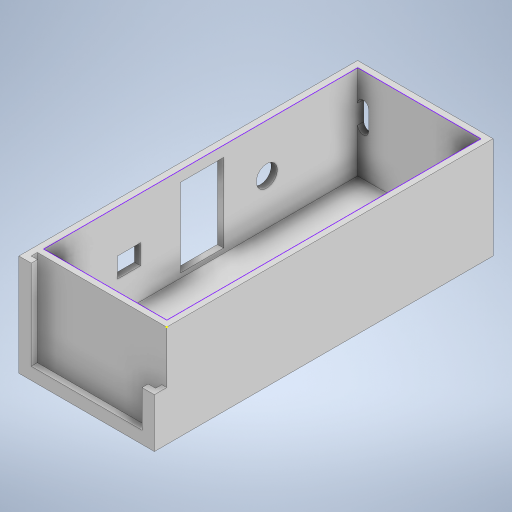
# Autodesk Inventor part: roller_box_new03_10_2025
Saved by Autodesk Inventor 2024.2 (Build 282272000, 272)
## iProperties
Created: 2025-08-30
Part Number: roller_box_new03_10_2025
Material: Типовые
Document SubType Name: Modeling
Designer: winds
Density: 1 g/cm^3
Appearance: По умолчанию
Author: winds
Autodesk Inventor part; units mm, degrees
ref_plane "YZ Plane" through (0, 0, 0) normal (1, 0, 0) x (0, 1, 0)
ref_plane "XZ Plane" through (0, 0, 0) normal (0, 1, 0) x (-1, 0, 0)
ref_plane "XY Plane" through (0, 0, 0) normal (0, 0, 1) x (1, 0, 0)
sketch "внешние размеры" plane through (0, 0, 0) normal (0, 1, 0) x (-1, 0, 0)
  line L0 (0, 0) -> (44, 0)
  line L1 (44, 0) -> (44, -106)
  line L2 (44, -106) -> (0, -106)
  line L3 (0, -106) -> (0, 0)
  dimension "d0" = 44
  dimension "d1" = 106
  constraints: 8 end point, 2 parallel, 1 horizontal, 1 perpendicular
  measures "d0" distance of L0.start L0.end
  measures "d1" distance between parallel lines of L0 L2
extrude "Выдавливание1" add sketch "внешние размеры" along normal blind 33
sketch "внутренние размеры" plane through (0, 33, 0) normal (0, 1, 0) x (1, 0, 0)
  line L0 (-42, 2) -> (-2, 2)
  line L1 (-2, 2) -> (-2, 104)
  line L2 (-2, 104) -> (-42, 104)
  line L3 (-42, 104) -> (-42, 2)
  point P0 (0, 0)
  constraints: 8 end point, 2 parallel, 1 horizontal, 1 perpendicular
extrude "Выдавливание2" cut sketch "внутренние размеры" against normal blind 30.5
sketch "перегородка" plane through (0, 2.5, 0) normal (0, 1, 0) x (1, 0, 0)
  line L0 (-42, 104) -> (-2, 104) projected
  line L1 (-20.5, 104) -> (-21.5, 104)
  line L2 (-21.5, 104) -> (-21.5, 54)
  line L3 (-21.5, 54) -> (-20.5, 54)
  line L4 (-20.5, 54) -> (-20.5, 104)
  line L5 (-2, 104) -> (-2, 2) projected
  line L6 (-42, 104) -> (-2, 104) projected
  point P0 (0, 0)
  point P1 (-22, 104)
  point P2 (-21, 54)
  dimension "d6" = 18.5
  dimension "d7" = 1
  dimension "d8" = 50
  constraints: 8 end point, 2 midpoint, 2 parallel, 1 horizontal, 1 perpendicular, 1 point on line
  measures "d6" distance between parallel lines of L4 L5
  measures "d7" distance between parallel lines of L4 L2
  measures "d8" vertical distance of point (-22, 104) point (-21, 54)
extrude "Выдавливание3" add sketch "перегородка" along normal blind 10
sketch "дисплей" plane through (-44, 0, -106) normal (-1, 0, 0) x (0, 0, 1)
  line L0 (45.5, 4) -> (59.5, 4)
  line L1 (59.5, 4) -> (59.5, 29.5)
  line L2 (59.5, 29.5) -> (45.5, 29.5)
  line L3 (45.5, 29.5) -> (45.5, 4)
  line L4 (0, 0) -> (0, 33) projected
  line L5 (0, 0) -> (106, 0) projected
  line L6 (0, 33) -> (106, 33) projected
  point P0 (0, 16.5)
  point P1 (59.5, 16.75)
  dimension "d21" = 25.5
  dimension "d22" = 14
  dimension "d23" = 45.5
  dimension "d24" = 4
  dimension "d25" = 3.5
  dimension "d125" = 59.5
  constraints: 8 end point, 2 midpoint, 2 parallel, 1 horizontal, 1 perpendicular
  measures "d21" distance of L2.end L0.start
  measures "d22" distance of L1.end L2.end
  measures "d23" distance between parallel lines of L4 L3
  measures "d24" distance between parallel lines of L5 L0
  measures "d25" distance between parallel lines of L6 L2
  measures "d125" horizontal distance of point (0, 16.5) point (59.5, 16.75)
extrude "Выдавливание4" cut sketch "дисплей" against normal blind 2.5
sketch "уф" plane through (-44, 0, -106) normal (-1, 0, 0) x (0, 0, 1)
  line L0 (80, 12.5) -> (72.5, 12.5)
  line L1 (72.5, 12.5) -> (72.5, 19)
  line L2 (72.5, 19) -> (80, 19)
  line L3 (80, 19) -> (80, 12.5)
  line L4 (106, 0) -> (106, 33) projected
  line L5 (0, 0) -> (106, 0) projected
  line L6 (0, 33) -> (106, 33) projected
  line L7 (0, 0) -> (0, 33) projected
  point P0 (80, 15.75)
  point P1 (72.5, 15.75)
  point P2 (0, 16.5)
  dimension "d28" = 7.5
  dimension "d29" = 6.5
  dimension "d30" = 26
  dimension "d31" = 12.5
  dimension "d32" = 14
  dimension "d126" = 72.5
  constraints: 8 end point, 3 midpoint, 2 parallel, 1 horizontal, 1 perpendicular
  measures "d28" distance of point (80, 15.75) point (72.5, 15.75)
  measures "d29" distance between parallel lines of L2 L0
  measures "d30" distance between parallel lines of L4 L3
  measures "d31" distance between parallel lines of L5 L0
  measures "d32" distance between parallel lines of L6 L2
  measures "d126" horizontal distance of point (0, 16.5) L1.end
extrude "Выдавливание5" cut sketch "уф" against normal blind 2.5 contours L0 L1 L2 L3
sketch "usb-c" plane through (0, 0, -106) normal (0, 0, -1) x (-1, 0, 0)
  line L0 (40.2, 24.8) -> (40.2, 15) construction
  line L1 (42, 4) -> (42, 29.5) projected
  line L2 (42, 23) -> (42, 16.8)
  line L3 (38.4, 16.8) -> (38.4, 23)
  arc A0 (42, 23) -> (38.4, 23) centre (40.2, 23) ccw
  arc A1 (38.4, 16.8) -> (42, 16.8) centre (40.2, 16.8) ccw
  line L4 (44, 0) -> (44, 33) projected
  line L5 (0, 0) -> (44, 0) projected
  point P0 (40.2, 19.9)
  point P1 (42, 19.9)
  point P2 (38.4, 19.9)
  point P3 (42, 16.8)
  point P4 (42, 23)
  dimension "d35" = 2
  dimension "d36" = 15
  dimension "d37" = 9.8
  dimension "d38" = 3.6
  constraints: 8 end point, 8 point on circle, 4 tangent, 3 midpoint, 2 centre point, 2 parallel, 2 point on line
  measures "d35" distance from line of L4 point (42, 19.9)
  measures "d36" distance from line of L5 point (40.2, 15)
  measures "d37" distance of point (40.2, 24.8) L0.end
  measures "d38" distance of point (38.4, 19.9) point (42, 19.9)
extrude "Выдавливание6" cut sketch "usb-c" against normal blind 2.5
sketch "stepper уши" plane through (0, 2.5, 0) normal (0, 1, 0) x (1, 0, 0)
  line L0 (-42, 2) -> (-42, 104) projected
  line L1 (-2, 2) -> (-42, 2) projected
  point P0 (0, 0)
  point P1 (-38.5, 5.5)
  point P2 (-15.5, 32)
  point P3 (-33, 24)
  point P4 (-33, 24)
  dimension "d41" = 3.5
  dimension "d42" = 3.5
  dimension "d43" = 26.5
  dimension "d44" = 30
  dimension "d45" = 35.0892
  dimension "d46" = 22
  dimension "d47" = 9
  dimension "d48" = 19.2419
  dimension "d49" = 19.3003
  constraints: 1 coincident
  measures "d41" distance from line of L0 point (-38.5, 5.5)
  measures "d42" distance from line of L1 point (-38.5, 5.5)
  measures "d43" distance from line of L0 point (-15.5, 32)
  measures "d44" distance from line of L1 point (-15.5, 32)
  measures "d45" distance of point (-15.5, 32) point (-38.5, 5.5)
  measures "d46" distance from line of L1 point (-33, 24)
  measures "d47" distance from line of L0 point (-33, 24)
  measures "d48" distance of point (-15.5, 32) point (-33, 24)
  measures "d49" distance of point (-33, 24) point (-38.5, 5.5)
hole "Отверстие2" at (-33, 2.5, -24) at (-15.5, 2.5, -32) at (-38.5, 2.5, -5.5) at (-33, 2.5, -24) direction (0, -1, 0) diameter 2.5 depth 2.5 tip angle 118
sketch "stepper ось" plane through (0, 2.5, 0) normal (0, 1, 0) x (1, 0, 0)
  circle A0 centre (-33, 24) radius 1.25 projected
  line L0 (-44, 0) -> (0, 0) projected
  line L1 (0, 0) -> (0, 106) projected
  dimension "d127" = 24
  dimension "d128" = 33
  constraints: 1 coincident
  measures "d127" distance from line of L0 point (-33, 24)
  measures "d128" distance from line of L1 point (-33, 24)
hole "Отверстие3" at (-33, 2.5, -24) direction (0, -1, 0) diameter 10 depth 2.5 tip angle 118
sketch "solar" plane through (0, 2.5, 0) normal (0, 1, 0) x (1, 0, 0)
  line L0 (-2, 104) -> (-2, 2) projected
  line L1 (-2, 2) -> (-8, 2)
  line L2 (-8, 2) -> (-8, 9.5)
  line L3 (-8, 9.5) -> (-2, 9.5)
  line L4 (-2, 9.5) -> (-2, 2)
  point P0 (0, 0)
  point P1 (-5, 2)
  point P2 (-5, 9.5)
  point P3 (-2, 9.5)
  dimension "d64" = 6
  dimension "d65" = 7.5
  constraints: 8 end point, 2 midpoint, 2 parallel, 1 horizontal, 1 perpendicular
  measures "d64" distance between parallel lines of L0 L2
  measures "d65" distance of point (-5, 2) point (-5, 9.5)
extrude "Выдавливание7" cut sketch "solar" against normal blind 2.5
sketch "кнопка" plane through (-44, 0, -106) normal (-1, 0, 0) x (0, 0, 1)
  line L0 (0, 0) -> (106, 0) projected
  line L1 (0, 0) -> (0, 33) projected
  point P0 (31.5, 17.3)
  dimension "d116" = 17.3
  dimension "d117" = 31.5
  measures "d116" distance from line of L0 point (31.5, 17.3)
  measures "d117" distance from line of L1 point (31.5, 17.3)
hole "Отверстие7" at (-44, 17.3, -74.5) direction (1, 0, 0) diameter 6.9 depth 2.5 tip angle 118
sketch "Эскиз25" plane through (-44, 0, -106) normal (-1, 0, 0) x (0, 0, 1)
  line L0 (106, 0) -> (106, 33) projected
  line L1 (106, 33) -> (110, 33)
  line L2 (110, 33) -> (110, 0)
  line L3 (110, 0) -> (106, 0)
  line L4 (106, 0) -> (106, 33)
  constraints: 8 end point, 2 parallel, 1 horizontal, 1 perpendicular
extrude "Выдавливание12" add sketch "Эскиз25" against normal blind 44
sketch "паз" plane through (-44, 0, -106) normal (-1, 0, 0) x (0, 0, 1)
  line L0 (106, 33) -> (108, 33)
  line L1 (108, 33) -> (108, 2)
  line L2 (108, 2) -> (106, 2)
  line L3 (106, 2) -> (106, 33)
  line L4 (110, 33) -> (110, 0) projected
  line L5 (108, 33) -> (110, 33)
  line L6 (110, 33) -> (110, 4)
  line L7 (110, 4) -> (108, 4)
  line L8 (108, 4) -> (108, 33)
  point P0 (106, 0)
  point P1 (107, 2)
  point P2 (107, 33)
  point P3 (109, 4)
  point P4 (109, 33)
  dimension "d133" = 31
  dimension "d134" = 29
  dimension "d135" = 2
  constraints: 16 end point, 4 midpoint, 4 parallel, 2 horizontal, 2 perpendicular, 2 point on line
  measures "d133" distance of point (107, 2) point (107, 33)
  measures "d134" distance of point (109, 4) point (109, 33)
  measures "d135" distance between parallel lines of L1 L3
extrude "Выдавливание13" cut sketch "паз" against normal blind 44
sketch "Эскиз27" plane through (0, 2.5, 0) normal (0, 1, 0) x (1, 0, 0)
  line L0 (-42, 104) -> (-2, 104) projected
  line L1 (-18, 60) -> (-17, 60)
  line L2 (-17, 60) -> (-17, 104)
  line L3 (-17, 104) -> (-18, 104)
  line L4 (-18, 104) -> (-18, 60)
  point P0 (0, 0)
  constraints: 8 end point, 2 parallel, 1 horizontal, 1 perpendicular, 1 point on line
extrude "Выдавливание14" add sketch "Эскиз27" along normal blind 3 draft -10
sketch "Эскиз28" plane through (0, 2.5, 0) normal (0, 1, 0) x (1, 0, 0)
  line L0 (-2, 104) -> (-2, 2) projected
  line L1 (-2, 18) -> (-10, 18)
  line L2 (-10, 18) -> (-10, 19)
  line L3 (-10, 19) -> (-2, 19)
  line L4 (-2, 19) -> (-2, 18)
  line L5 (-2, 104) -> (-2, 9.5) projected
  line L6 (-2, 27) -> (-10, 27)
  line L7 (-10, 27) -> (-10, 28)
  line L8 (-10, 28) -> (-2, 28)
  line L9 (-2, 28) -> (-2, 27)
  line L10 (-10, 28) -> (-11, 28)
  line L11 (-11, 28) -> (-11, 18)
  line L12 (-11, 18) -> (-10, 18)
  line L13 (-10, 18) -> (-10, 28)
  point P0 (0, 0)
  point P1 (-2, 19)
  constraints: 24 end point, 6 parallel, 3 horizontal, 3 perpendicular, 3 point on line
extrude "Выдавливание15" add sketch "Эскиз28" along normal blind 13.5 contours L0 L6 L7 L8 | L7 L13 L2 L12 L11 L10 | L0 L1 L2 L3
sketch "кнопка2" plane through (0, 2.5, 0) normal (0, 1, 0) x (1, 0, 0)
  circle A0 centre (-6, 23) radius 3.6
  line L0 (0, -4) -> (0, 106) projected
  line L1 (-2, 19) -> (-10, 19) projected
  point P0 (0, 0)
  dimension "d147" = 7.2
  dimension "d172" = 6
  dimension "d173" = 4
  constraints: 1 centre point
  measures "d147" diameter of A0
  measures "d172" distance from line of L0 A0.centre
  measures "d173" distance from line of A0.centre L1
hole "Отверстие9" at (-6, 2.5, -23) direction (0, -1, 0) diameter 7.2 depth 2.5 tip angle 118
sketch "Эскиз31" plane through (0, 2.5, 0) normal (0, 1, 0) x (1, 0, 0)
  line L0 (-2, 104) -> (-2, 2) projected
  line L1 (-2, 2) -> (-42, 2) projected
  line L2 (-2, 10) -> (-3, 10)
  line L3 (-3, 10) -> (-3, 2)
  line L4 (-3, 2) -> (-2, 2)
  line L5 (-2, 2) -> (-2, 10)
  point P0 (0, 0)
  constraints: 8 end point, 2 parallel, 2 point on line, 1 horizontal, 1 perpendicular
extrude "Выдавливание16" add sketch "Эскиз31" along normal blind 2
sketch "Эскиз32" plane through (-44, 4, 4) normal (0, 1, 0) x (1, 0, 0)
  line L0 (0, 0) -> (44, 0) projected
  line L1 (44, 4) -> (40, 4)
  line L2 (40, 0) -> (44, 0)
  line L3 (44, 0) -> (44, 4)
  line L4 (0, 110) -> (0, 0) projected
  line L5 (0, 4) -> (44, 4) projected
  line L6 (0, 0) -> (4, 0)
  line L7 (4, 0) -> (4, 4)
  line L8 (4, 4) -> (0, 4)
  line L9 (0, 4) -> (0, 0)
  point P0 (4, 0)
  constraints: 14 end point, 3 parallel, 2 horizontal, 2 point on line, 1 perpendicular
extrude "Выдавливание17" add sketch "Эскиз32" along normal blind 29 contours L4 L5 L7 L0
sketch "Эскиз33" plane through (0, 4, 4) normal (0, 1, 0) x (1, 0, 0)
  line L0 (0, 4) -> (-4, 4)
  line L1 (-4, 4) -> (-4, 0)
  line L2 (-4, 0) -> (0, 0)
  line L3 (0, 0) -> (0, 4)
  constraints: 8 end point, 2 parallel, 1 horizontal, 1 perpendicular
extrude "Выдавливание18" add sketch "Эскиз33" along normal blind 12
sketch "Эскиз34" plane through (0, 16, 4) normal (0, 1, 0) x (1, 0, 0)
  line L0 (-44, 2) -> (0, 2) projected
  line L1 (-40, 4) -> (0, 4) projected
  line L2 (-1.6, 2) -> (-4, 2)
  line L3 (-4, 2) -> (-4, 4)
  line L4 (-4, 4) -> (-1.6, 4)
  line L5 (-1.6, 4) -> (-1.6, 2)
  line L6 (-40, 2) -> (-42, 2)
  line L7 (-42, 2) -> (-42, 4)
  line L8 (-42, 4) -> (-40, 4)
  line L9 (-40, 4) -> (-40, 2)
  point P0 (-1.6, 4)
  point P1 (-4, 2)
  point P2 (-1.6, 3)
  point P3 (-4, 3)
  point P4 (-2.8, 2)
  point P5 (-2.8, 4)
  dimension "d169" = 2.4
  dimension "d170" = 2
  constraints: 16 end point, 4 midpoint, 4 parallel, 4 point on line, 2 horizontal, 2 perpendicular
  measures "d169" distance of point (-1.6, 3) point (-4, 3)
  measures "d170" distance of point (-2.8, 2) point (-2.8, 4)
extrude "Выдавливание19" cut sketch "Эскиз34" against normal blind 15 contours L3 L1 L5 L0
sketch "Эскиз35" plane through (0, 33, 0) normal (0, 1, 0) x (1, 0, 0)
  line L0 (-40, -2) -> (-4, -2) projected
  line L1 (-40, 0) -> (-44, 0) projected
  line L2 (-40, -2) -> (-42, -2)
  line L3 (-42, -2) -> (-42, 0)
  line L4 (-42, 0) -> (-40, 0)
  line L5 (-40, 0) -> (-40, -2)
  point P0 (0, 0)
  point P1 (-40, -1)
  point P2 (-42, -1)
  dimension "d171" = 2
  constraints: 8 end point, 3 midpoint, 2 parallel, 1 horizontal, 1 perpendicular
  measures "d171" distance of point (-40, -1) point (-42, -1)
extrude "Выдавливание20" cut sketch "Эскиз35" against normal blind 31
sketch "Эскиз36" plane through (-44, 0, -106) normal (-1, 0, 0) x (0, 0, 1)
  line L0 (108, 33) -> (108, 4) projected
  line L1 (106, 2) -> (108, 2) projected
  line L2 (108, 4) -> (106, 4)
  line L3 (106, 4) -> (106, 2)
  line L4 (106, 2) -> (108, 2)
  line L5 (108, 2) -> (108, 4)
  point P0 (106, 0)
  constraints: 8 end point, 2 parallel, 1 horizontal, 1 perpendicular
extrude "Выдавливание21" add sketch "Эскиз36" against normal blind 2
sketch "Эскиз37" plane through (0, 0, -106) normal (1, 0, 0) x (0, 0, -1)
  line L0 (-108, 2) -> (-108, 4) projected
  line L1 (-106, 4) -> (-106, 2) projected
  line L2 (-108, 4) -> (-106, 4)
  line L3 (-106, 4) -> (-106, 2)
  line L4 (-106, 2) -> (-108, 2)
  line L5 (-108, 2) -> (-108, 4)
  point P0 (-106, 0)
  constraints: 8 end point, 2 parallel, 1 horizontal, 1 perpendicular
extrude "Выдавливание22" add sketch "Эскиз37" against normal blind 2
